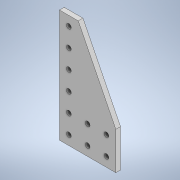
# Autodesk Inventor part: 6x3
Saved by Autodesk Inventor 2020 (Build 240168000, 168)
## iProperties
Created: 2020-01-13
Part Number: 6x3
Material: Generic
Document SubType Name: Modeling
Designer: 339294
Density: 1 g/cm^3
Appearance: Default
Author: 339294
Autodesk Inventor part; units mm, degrees
ref_plane "YZ Plane" through (0, 0, 0) normal (1, 0, 0) x (0, 1, 0)
ref_plane "XZ Plane" through (0, 0, 0) normal (0, 1, 0) x (-1, 0, 0)
ref_plane "XY Plane" through (0, 0, 0) normal (0, 0, 1) x (1, 0, 0)
sketch "Sketch1" plane through (0, 0, 0) normal (0, 0, 1) x (1, 0, 0)
  line L0 (0, 0) -> (76.2, 0)
  line L1 (76.2, 0) -> (76.2, 50.8)
  line L2 (0, 50.8) -> (0, 0)
  line L3 (25.4, 152.4) -> (0, 152.4)
  line L4 (0, 152.4) -> (0, 50.8)
  line L5 (25.4, 152.4) -> (76.2, 50.8)
  circle A0 centre (12.7, 12.7) radius 3.2512
  circle A1 centre (12.7, 38.1) radius 3.2512
  circle A2 centre (12.7, 63.5) radius 3.2512
  circle A3 centre (12.7, 88.9) radius 3.2512
  circle A4 centre (12.7, 114.3) radius 3.2512
  circle A5 centre (12.7, 139.7) radius 3.2512
  circle A6 centre (38.1, 12.7) radius 3.2512
  circle A7 centre (63.5, 12.7) radius 3.2512
  circle A8 centre (12.7, 38.1) radius 3.2512
  circle A9 centre (38.1, 38.1) radius 3.2512
  circle A10 centre (63.5, 38.1) radius 3.2512
  dimension "d4" = 101.6
  dimension "d5" = 50.8
  dimension "d6" = 25.4
  dimension "d7" = 50.8
  dimension "d8" = 101.6
  dimension "d9" = 50.8
  dimension "d10" = 76.2
  dimension "d11" = 6.5024
  dimension "d12" = 12.7
  dimension "d13" = 12.7
  dimension "d16" = 25.4
  dimension "d23" = 25.4
  dimension "d26" = 25.4
  constraints: 12 end point, 11 centre point, 2 horizontal, 2 vertical, 1 parallel, 1 perpendicular, 20 other
  measures "d4" distance of L3.end L2.start
  measures "d5" distance of L2.start L0.start
  measures "d6" distance of L3.start L3.end
  measures "d7" horizontal distance of L3.start L1.end
  measures "d8" vertical distance of L3.start L1.end
  measures "d9" distance of L0.end L1.end
  measures "d10" distance of L0.start L0.end
  measures "d11" diameter of A0
  measures "d12" distance from line of L0 A0.centre
  measures "d13" distance from line of L2 A0.centre
  measures "d16" distance of A0.centre A1.centre
  measures "d23" distance of A0.centre A6.centre
  measures "d26" distance of A0.centre A8.centre
extrude "Extrusion1" add sketch "Sketch1" along normal blind 6.35
body "Solid1"
